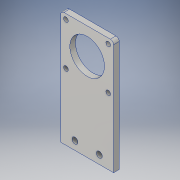
# Autodesk Inventor part: Motor Support
Saved by Autodesk Inventor 2016 (Build 200138000, 138)
## iProperties
Created: 2015-06-02
Part Number: Motor Support
Material: Aluminum 6061
Document SubType Name: Modeling
Designer: Dennis
Density: 2.7 g/cm^3
Appearance: Aluminum - Flat
Mass: 103.218 g
Surface Area: 158.034 cm^2
Volume: 38.2291 cm^3
Author: Dennis
Autodesk Inventor part; units mm, degrees
ref_plane "YZ Plane" through (0, 0, 0) normal (1, 0, 0) x (0, 1, 0)
ref_plane "XZ Plane" through (0, 0, 0) normal (0, 1, 0) x (-1, 0, 0)
ref_plane "XY Plane" through (0, 0, 0) normal (0, 0, 1) x (1, 0, 0)
sketch "Sketch1" plane through (0, 0, 0) normal (0, 0, 1) x (1, 0, 0)
  line L0 (0, 0) -> (58.8772, 0)
  line L1 (58.8772, 0) -> (58.8772, 127)
  line L2 (58.8772, 127) -> (0, 127)
  line L3 (0, 127) -> (0, 0)
  dimension "d0" = 58.8772
  dimension "d1" = 127
  constraints: 8 end point, 2 parallel, 1 horizontal, 1 perpendicular
  measures "d0" distance of L0.start L0.end
  measures "d1" distance of L2.end L0.start
extrude "Extrusion1" add sketch "Sketch1" along normal blind 6.35
sketch "Sketch2" plane through (0, 0, 6.35) normal (0, 0, 1) x (1, 0, 0)
  circle A0 centre (29.4386, 97.5614) radius 19.304
  line L0 (58.8772, 127) -> (0, 127) projected
  line L1 (0, 127) -> (0, 0) projected
  line L2 (58.8772, 0) -> (58.8772, 127) projected
  line L3 (29.4386, 127) -> (29.4386, 0)
  line L4 (0, 0) -> (58.8772, 0) projected
  dimension "d4" = 38.608
  dimension "d5" = 29.4386
  constraints: 2 end point, 2 midpoint, 1 centre point, 1 point on line
  measures "d4" diameter of A0
  measures "d5" distance from line of L0 A0.centre
extrude "Extrusion2" cut sketch "Sketch2" against normal blind 6.35 contours A0 L3 | L3 A0
sketch "Sketch3" plane through (0, 0, 6.35) normal (0, 0, 1) x (1, 0, 0)
  circle A0 centre (5.8166, 121.1834) radius 2.6035
  line L0 (58.8772, 127) -> (0, 127) projected
  line L1 (0, 127) -> (0, 0) projected
  circle A1 centre (5.8166, 74.041) radius 2.6035
  circle A2 centre (52.959, 121.1834) radius 2.6035
  circle A3 centre (52.959, 74.041) radius 2.6035
  dimension "d10" = 5.207
  dimension "d11" = 5.8166
  dimension "d12" = 5.8166
  dimension "d15" = 47.1424
  dimension "d18" = 47.1424
  constraints: 4 centre point, 1 horizontal, 1 vertical, 6 other
  measures "d10" diameter of A0
  measures "d11" distance from line of A0.centre L0
  measures "d12" distance from line of A0.centre L1
  measures "d15" distance of A0.centre A1.centre
  measures "d18" distance of A0.centre A2.centre
extrude "Extrusion3" cut sketch "Sketch3" against normal blind 6.35
fillet "Fillet1" radius 3.6068 2 edges at (0, 127, 3.175) (58.8772, 127, 3.175)
sketch "Sketch4" plane through (0, 0, 6.35) normal (0, 0, 1) x (1, 0, 0)
  circle A0 centre (15.875, 9.525) radius 3.302
  circle A1 centre (43.0022, 9.525) radius 3.302
  line L0 (0, 0) -> (58.8772, 0) projected
  line L1 (58.8772, 0) -> (58.8772, 123.3932) projected
  line L2 (0, 123.3932) -> (0, 0) projected
  dimension "d24" = 6.604
  dimension "d25" = 6.604
  dimension "d26" = 9.525
  dimension "d27" = 9.525
  dimension "d28" = 15.875
  dimension "d29" = 15.875
  constraints: 2 centre point
  measures "d24" diameter of A0
  measures "d25" diameter of A1
  measures "d26" distance from line of A0.centre L0
  measures "d27" distance from line of A1.centre L0
  measures "d28" distance from line of A1.centre L1
  measures "d29" distance from line of A0.centre L2
extrude "Extrusion4" cut sketch "Sketch4" against normal blind 25.4
body "Solid1"
